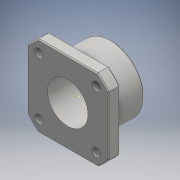
# Autodesk Inventor part: 608ZZ Ball Screw Support Unit
Saved by Autodesk Inventor 2016 (Build 200138000, 138)
## iProperties
Created: 2017-07-18
Part Number: 608ZZ Ball Screw Support Unit
Material: Generic
Document SubType Name: Modeling
Designer: M228544
Density: 1 g/cm^3
Appearance: Default
Author: M228544
Autodesk Inventor part; units mm, degrees
ref_plane "YZ Plane" through (0, 0, 0) normal (1, 0, 0) x (0, 1, 0)
ref_plane "XZ Plane" through (0, 0, 0) normal (0, 1, 0) x (-1, 0, 0)
ref_plane "XY Plane" through (0, 0, 0) normal (0, 0, 1) x (1, 0, 0)
sketch "Sketch1" plane through (0, 0, 0) normal (0, 1, 0) x (-1, 0, 0)
  line L0 (21, -21) -> (-21, -21)
  line L1 (-21, -21) -> (-21, 21)
  line L2 (-21, 21) -> (21, 21)
  line L3 (21, 21) -> (21, -21)
  point P0 (0, 0)
  dimension "d3" = 42
  dimension "d4" = 42
  constraints: 8 end point, 2 parallel, 1 horizontal, 1 perpendicular
  measures "d3" distance of L1.end L2.end
  measures "d4" distance of L0.end L1.end
extrude "Extrusion1" add sketch "Sketch1" along normal blind 6
sketch "Sketch2" plane through (0, 6, 0) normal (0, 1, 0) x (1, 0, 0)
  circle A0 centre (0, 0) radius 16.95
  dimension "d7" = 33.9
  constraints: 1 centre point, 1 coincident
  measures "d7" diameter of A0
extrude "Extrusion2" add sketch "Sketch2" along normal blind 17.1
sketch "Sketch3" plane through (0, 23.1, 0) normal (0, 1, 0) x (1, 0, 0)
  circle A0 centre (0, 0) radius 10.5
  dimension "d10" = 21
  constraints: 1 centre point, 1 coincident
  measures "d10" diameter of A0
extrude "Extrusion3" cut sketch "Sketch3" against normal blind 76.65
sketch "Sketch4" plane through (0, 6, 0) normal (0, 1, 0) x (1, 0, 0)
  point P0 (0, 0)
sketch "Sketch5" plane through (0, 0, 0) normal (0, -1, 0) x (1, 0, 0)
  line L0 (-21, -21) -> (21, -21) projected
  circle A0 centre (0, 0) radius 10.5 projected
  line L1 (-21, -21) -> (0, 0)
  line L2 (-7.4246, -7.4246) -> (-12.0208, -12.0208)
  line L3 (-12.0208, -12.0208) -> (-17.6777, -17.6777)
  circle A1 centre (-14.8492, -14.8492) radius 4
  circle A2 centre (-14.8492, -14.8492) radius 2.25
  circle A3 centre (14.8492, -14.8492) radius 2.25
  circle A4 centre (14.8492, 14.8492) radius 2.25
  circle A5 centre (-14.8492, 14.8492) radius 2.25
  dimension "d13" = 6.5
  dimension "d14" = 8
  dimension "d15" = 4.5
  dimension "d18" = 360
  constraints: 6 end point, 4 centre point, 3 point on line, 1 coincident, 1 midpoint, 14 other
  measures "d13" distance of L2.start L2.end
  measures "d14" distance of L2.end L3.end
  measures "d15" diameter of A2
extrude "Extrusion4" cut sketch "Sketch5" against normal blind 88.15 contours A2 L1 | L1 A2 | A3 | A4 | A5
chamfer "Chamfer1" distance 1 angle 45 1 edges at (-16.95, 23.1, 0)
chamfer "Chamfer2" distance 0.5 angle 45 4 edges at (0, 6, -21) (-21, 6, 0) (0, 6, 21) (21, 6, 0)
sketch "Sketch6" plane through (0, 6, 0) normal (0, 1, 0) x (1, 0, 0)
  line L0 (-20.5, -20.5) -> (-20.5, 20.5) projected
  circle A0 centre (0, 0) radius 15.95 projected
  line L1 (-20.5, 20.5) -> (0, 0)
  circle A1 centre (0, 0) radius 10.5 projected
  line L2 (-7.4246, 7.4246) -> (-18.3848, 18.3848)
  circle A2 centre (0, 0) radius 26
  circle A3 centre (0, 0) radius 31.7761
  dimension "d28" = 15.5
  constraints: 4 end point, 2 coincident, 2 point on line, 1 centre point, 5 other
  measures "d28" distance of L2.start L2.end
extrude "Extrusion5" cut sketch "Sketch6" against normal blind 219.6 contours L0 L1 A2 | A3
chamfer "Chamfer3" distance 0.5 angle 45 12 edges at (-18.3848, 6, -18.3848) (18.3848, 6, -18.3848) (18.3848, 6, 18.3848) (-18.3848, 6, 18.3848) (-18.3848, 0, -18.3848) (0, 0, -21) (18.3848, 0, -18.3848) (21, 0, 0) (18.3848, 0, 18.3848) (0, 0, 21) (-18.3848, 0, 18.3848) (-21, 0, 0)
body "Solid1"
